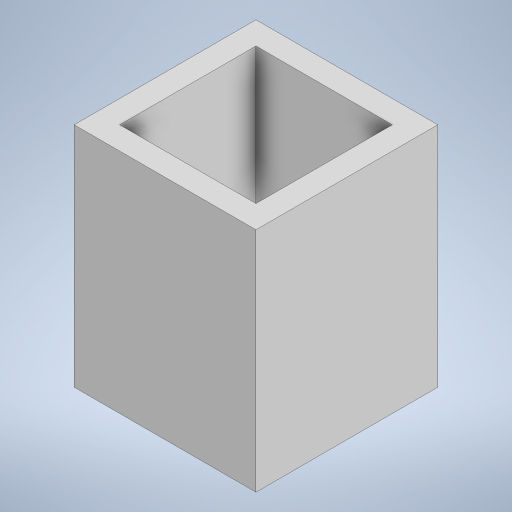
# Autodesk Inventor part: battery5V_box
Saved by Autodesk Inventor 2023 (Build 270158000, 158)
## iProperties
Created: 2023-05-22
Part Number: battery5V_box
Material: 一般
Document SubType Name: Modeling
Designer: 310611102
Density: 1 g/cm^3
Appearance: 預設
Author: 310611102
Autodesk Inventor part; units mm, degrees
ref_plane "YZ Plane" through (0, 0, 0) normal (1, 0, 0) x (0, 1, 0)
ref_plane "XZ Plane" through (0, 0, 0) normal (0, 1, 0) x (-1, 0, 0)
ref_plane "XY Plane" through (0, 0, 0) normal (0, 0, 1) x (1, 0, 0)
sketch "Sketch1" plane through (0, 0, 0) normal (0, 0, 1) x (1, 0, 0)
  line L0 (0, 0) -> (-40, 0)
  line L1 (-40, 0) -> (-40, 50)
  line L2 (-40, 50) -> (0, 50)
  line L3 (0, 50) -> (0, 0)
  dimension "d0" = 50
  dimension "d1" = 40
  constraints: 8 end point, 2 parallel, 1 horizontal, 1 perpendicular
  measures "d0" distance of L2.end L0.start
  measures "d1" distance of L1.end L2.end
extrude "Extrusion1" add sketch "Sketch1" along normal blind 40
sketch "Sketch2" plane through (-40, 50, 0) normal (0, 1, 0) x (1, 0, 0)
  line L0 (40, 0) -> (0, 0) projected
  line L1 (0, 0) -> (0, -40) projected
  line L2 (40, -40) -> (0, -40) projected
  line L3 (40, 0) -> (40, -40) projected
  line L4 (5, -5) -> (35, -5)
  line L5 (35, -5) -> (35, -35)
  line L6 (35, -35) -> (5, -35)
  line L7 (5, -35) -> (5, -5)
  dimension "d5" = 5
  constraints: 8 end point, 3 other
  measures "d5" distance between parallel lines of L0 L4
extrude "Extrusion2" cut sketch "Sketch2" against normal blind 30 contours L4 L5 L6 L7
sketch "Sketch3" plane through (-40, 0, 0) normal (0, -1, 0) x (1, 0, 0)
  circle A0 centre (5, 35) radius 2.5
  line L0 (5, 35) -> (7.3437, 35)
  line L1 (7.3437, 35) -> (7.3437, 32.7108)
  circle A1 centre (35, 35) radius 2.5
  circle A2 centre (5, 5) radius 2.5
  circle A3 centre (35, 5) radius 2.5
  line L2 (0, 40) -> (40, 40) projected
  line L3 (0, 0) -> (0, 40) projected
  point P0 (40, 0)
  dimension "d10" = 30
  dimension "d13" = 30
  dimension "d16" = 5
  dimension "d17" = 5
  dimension "d18" = 5
  constraints: 4 centre point, 4 end point, 2 horizontal, 1 perpendicular, 1 vertical, 6 other
  measures "d10" distance of L0.start A1.centre
  measures "d13" distance of L0.start A2.centre
  measures "d16" diameter of A0
  measures "d17" distance from line of L2 L0.start
  measures "d18" distance from line of L3 L0.start
extrude "Extrusion3" cut sketch "Sketch3" against normal blind 10
body "Solid1"
